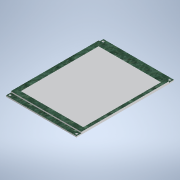
# Autodesk Inventor part: E-Paper Display
Saved by Autodesk Inventor 2020 (Build 240168000, 168)
## iProperties
Created: 2021-11-08
Part Number: E-Paper Display
Material: Generic
Document SubType Name: Modeling
Designer: mtkts
Density: 1 g/cm^3
Appearance: Default
Author: mtkts
Autodesk Inventor part; units mm, degrees
ref_plane "YZ Plane" through (0, 0, 0) normal (1, 0, 0) x (0, 1, 0)
ref_plane "XZ Plane" through (0, 0, 0) normal (0, 1, 0) x (-1, 0, 0)
ref_plane "XY Plane" through (0, 0, 0) normal (0, 0, 1) x (1, 0, 0)
sketch "Sketch1" plane through (0, 0, 0) normal (0, 1, 0) x (-1, 0, 0)
  line L0 (-50.22, 69.4) -> (50.22, 69.4)
  line L1 (50.22, 69.4) -> (50.22, -69.4)
  line L2 (50.22, -69.4) -> (-50.22, -69.4)
  line L3 (-50.22, -69.4) -> (-50.22, 69.4)
  line L4 (-50.22, 69.4) -> (50.22, -69.4) construction
  line L5 (50.22, 69.4) -> (-50.22, -69.4) construction
  point P0 (0, 0)
  dimension "d0" = 100.44
  dimension "d1" = 138.8
  constraints: 12 end point, 2 midpoint, 2 parallel, 1 horizontal, 1 perpendicular
  measures "d0" distance of L1.end L2.end
  measures "d1" distance of L0.end L1.end
extrude "Extrusion1" add sketch "Sketch1" along normal blind 1.75
sketch "Sketch2" plane through (0, 1.75, 0) normal (0, 1, 0) x (1, 0, 0)
  line L0 (-50.22, 69.4) -> (-50.22, -69.4) construction
  line L1 (50.22, -69.4) -> (50.22, 69.4) construction
  line L2 (50.22, -62.5) -> (-50.22, -62.5)
  line L3 (-50.22, -62.5) -> (-50.22, 62.5)
  line L4 (-50.22, 62.5) -> (50.22, 62.5)
  line L5 (50.22, 62.5) -> (50.22, -62.5)
  line L6 (50.22, -62.5) -> (-50.22, 62.5) construction
  line L7 (-50.22, -62.5) -> (50.22, 62.5) construction
  point P0 (0, 0)
  dimension "d4" = 125
  constraints: 12 end point, 2 midpoint, 2 parallel, 1 collinear, 1 perpendicular
  measures "d4" distance of L2.end L3.end
extrude "Extrusion2" add sketch "Sketch2" along normal blind 1.75
sketch "Sketch3" plane through (0, 1.75, 0) normal (0, 1, 0) x (1, 0, 0)
  line L0 (50.22, -62.5) -> (-50.22, -62.5) construction
  line L1 (-50.22, -62.5) -> (-50.22, -69.4) construction
  line L2 (-50.22, -69.4) -> (50.22, -69.4) construction
  line L3 (50.22, -69.4) -> (50.22, -62.5) construction
  line L4 (-50.22, 62.5) -> (50.22, 62.5) construction
  line L5 (50.22, 62.5) -> (50.22, 69.4) construction
  line L6 (50.22, 69.4) -> (-50.22, 69.4) construction
  line L7 (-50.22, 69.4) -> (-50.22, 62.5) construction
  line L8 (-50.22, -69.4) -> (50.22, -69.4) construction
  line L9 (0, -69.4) -> (0, 69.4) construction
  line L10 (50.22, 69.4) -> (-50.22, 69.4) construction
  line L11 (0, -66.25) -> (-47.5, -66.25) construction
  line L12 (0, -66.25) -> (47.5, -66.25) construction
  line L13 (-50.22, -62.5) -> (50.22, -62.5) construction
  line L14 (0, -66.25) -> (47.5, -66.25) construction
  circle A0 centre (-47.5, -66.25) radius 1.5
  circle A1 centre (47.5, -66.25) radius 1.5
  line L15 (-50.22, 69.4) -> (-50.22, -69.4) projected
  line L16 (-50.22, 0) -> (50.22, 0) construction
  line L17 (50.22, -62.5) -> (50.22, 62.5) projected
  circle A2 centre (-47.5, 66.25) radius 1.5
  circle A3 centre (47.5, 66.25) radius 1.5
  line L18 (50.22, -62.5) -> (-50.22, -62.5) projected
  line L19 (-50.22, -62.5) -> (-50.22, -69.4) projected
  line L20 (-50.22, -69.4) -> (50.22, -69.4) projected
  line L21 (50.22, -69.4) -> (50.22, -62.5) projected
  line L22 (-50.22, 62.5) -> (50.22, 62.5) projected
  line L23 (50.22, 69.4) -> (-50.22, 69.4) projected
  line L24 (50.22, 62.5) -> (50.22, 69.4) projected
  line L25 (-50.22, 69.4) -> (-50.22, 62.5) projected
  point P0 (0, 0)
  point P1 (-51, 62.5)
  dimension "d7" = 47.5
  dimension "d8" = 47.5
  dimension "d9" = 0
  dimension "d10" = 3
  dimension "d11" = 3
  constraints: 10 end point, 4 centre point, 3 midpoint, 2 coincident, 2 parallel, 2 symmetric about line, 1 collinear, 1 horizontal, 1 point on line, 4 other
  measures "d7" distance of L11.start L11.end
  measures "d8" distance of L11.start L12.end
  measures "d9" distance between parallel lines of L12 L14
  measures "d10" diameter of A0
  measures "d11" diameter of A1
extrude "Extrusion3" cut sketch "Sketch3" against normal through all contours A0 | A1 | A2 | A3
sketch "Sketch4" plane through (0, 0, 0) normal (0, -1, 0) x (1, 0, 0)
  circle A0 centre (47.5, -66.25) radius 1.5 construction
  circle A1 centre (-47.5, -66.25) radius 1.5 construction
  circle A2 centre (47.5, 66.25) radius 1.5 construction
  circle A3 centre (-47.5, 66.25) radius 1.5 construction
  line L0 (-50.22, 69.4) -> (50.22, 69.4) construction
  line L1 (-50.22, -69.4) -> (-50.22, 69.4) construction
  line L2 (50.22, -69.4) -> (-50.22, -69.4) construction
  line L3 (50.22, 69.4) -> (50.22, -69.4) construction
  circle A4 centre (-47.5, -66.25) radius 1.5 construction
  line L4 (50.22, -69.4) -> (8.97, -69.4) construction
  line L5 (50.22, -69.4) -> (-50.22, -69.4) construction
  line L6 (-50.22, -69.4) -> (-10.97, -69.4) construction
  line L7 (-10.97, -69.4) -> (-10.97, -61.4)
  line L8 (-10.97, -61.4) -> (9.03, -61.4)
  line L9 (9.03, -61.4) -> (9.03, -69.4)
  line L10 (9.03, -69.4) -> (-10.97, -69.4)
  point P0 (0, 0)
  dimension "d21" = 41.25
  dimension "d22" = 39.25
  dimension "d23" = 8
  dimension "d24" = 20
  constraints: 12 end point, 2 parallel, 2 point on line, 1 perpendicular, 1 vertical
  measures "d21" distance of L2.start L4.end
  measures "d22" distance of L1.start L6.end
  measures "d23" distance of L6.end L7.end
  measures "d24" distance of L7.end L8.end
extrude "Extrusion4" add sketch "Sketch4" along normal blind 6
sketch "Sketch5" plane through (0, 3.5, 0) normal (0, 1, 0) x (1, 0, 0)
  line L0 (50.22, 62.5) -> (-50.22, 62.5) construction
  line L1 (-50.22, 62.5) -> (-50.22, -62.5) construction
  line L2 (-50.22, -62.5) -> (50.22, -62.5) construction
  line L3 (50.22, -62.5) -> (50.22, 62.5) construction
  line L4 (-50.22, 62.5) -> (-50.22, -62.5) construction
  line L5 (-50.22, 62.5) -> (-50.22, 55.388) construction
  line L6 (-50.22, 55.388) -> (-43.108, 55.388) construction
  line L7 (50.22, 62.5) -> (50.22, 55.388) construction
  line L8 (50.22, -62.5) -> (50.22, 62.5) construction
  line L9 (50.22, 55.388) -> (41.33, 55.388) construction
  line L10 (-50.22, -62.5) -> (50.22, -62.5) construction
  line L11 (50.22, -62.5) -> (50.22, -55.388) construction
  line L12 (50.22, -55.388) -> (41.33, -55.388) construction
  line L13 (-50.22, -62.5) -> (-50.22, -69.4) construction
  line L14 (-50.22, -62.5) -> (-50.22, -55.388) construction
  line L15 (-50.22, -55.388) -> (-43.108, -55.388) construction
  line L16 (-43.108, 55.388) -> (45.775, 55.388)
  line L17 (45.775, 55.388) -> (45.775, -55.388)
  line L18 (45.775, -55.388) -> (-43.108, -55.388)
  line L19 (-43.108, -55.388) -> (-43.108, 55.388)
  point P0 (0, 0)
  dimension "d25" = 7.112
  dimension "d26" = 7.112
  dimension "d27" = 7.112
  dimension "d28" = 8.89
  dimension "d29" = 7.112
  dimension "d30" = 8.89
  dimension "d31" = 7.112
  dimension "d32" = 7.112
  constraints: 24 end point, 4 perpendicular, 4 point on line, 2 horizontal, 2 parallel, 1 midpoint
  measures "d25" distance of L0.end L5.end
  measures "d26" distance of L5.end L6.end
  measures "d27" distance of L0.start L7.end
  measures "d28" distance of L7.end L9.end
  measures "d29" distance of L2.end L11.end
  measures "d30" distance of L11.end L12.end
  measures "d31" distance of L1.end L14.end
  measures "d32" distance of L14.end L15.end
extrude "Extrusion5" add sketch "Sketch5" along normal blind 0.001
equation "\"d26\" = d25"
equation "\"d27\" = d25"
equation "\"d29\" = d25"
equation "\"d30\" = d28"
equation "\"d31\" = d25"
equation "\"d32\" = d25"
body "Solid1"
